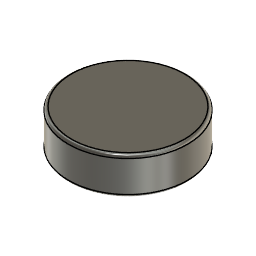
encoder_magnet_v1 (Autodesk Fusion 360 design; units mm, degrees)
Autodesk Fusion 360 part; units mm, degrees
sketch "Sketch1" plane through (0, 0, 0) normal (0, 0, 1) x (1, 0, 0)
  circle A0 centre (0, 0) radius 4
  dimension "d1" = 8
  constraint coincident A0.centre origin
  measures "d1" diameter of A0
extrude "Extrude1" add sketch "Sketch1" along normal blind 2.5
fillet "Fillet1" radius 0.2 1 edges at (-3.7293, -1.4465, 2.5)
fillet "Fillet2" radius 0.2 1 edges at (-3.7293, -1.4465, 0)
